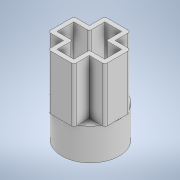
# Autodesk Inventor part: servo-axle-adapter-1-2
Saved by Autodesk Inventor 2020 (Build 240168000, 168)
## iProperties
Created: 2023-03-22
Part Number: servo-axle-adapter-1-2
Material: Generic
Document SubType Name: Modeling
Designer: 22hamfri
Density: 1 g/cm^3
Appearance: Default
Author: 22hamfri
Autodesk Inventor part; units mm, degrees
ref_plane "YZ Plane" through (0, 0, 0) normal (1, 0, 0) x (0, 1, 0)
ref_plane "XZ Plane" through (0, 0, 0) normal (0, 1, 0) x (-1, 0, 0)
ref_plane "XY Plane" through (0, 0, 0) normal (0, 0, 1) x (1, 0, 0)
sketch "Sketch1" plane through (0, 0, 0) normal (0, 1, 0) x (-1, 0, 0)
  circle A0 centre (0, 0) radius 2.6478
  line L0 (2.6478, 0) -> (2.4043, 0.3165)
  line L1 (2.6478, 0) -> (0, 0)
  line L2 (2.6478, 0) -> (2.4043, -0.3165)
  line L3 (2.5576, 0.6853) -> (2.2404, 0.928)
  line L4 (2.5576, 0.6853) -> (2.4043, 0.3165)
  line L5 (2.293, 1.3239) -> (1.9239, 1.4762)
  line L6 (2.293, 1.3239) -> (2.2404, 0.928)
  line L7 (1.8723, 1.8723) -> (1.4762, 1.9239)
  line L8 (1.8723, 1.8723) -> (1.9239, 1.4762)
  line L9 (1.3239, 2.293) -> (0.928, 2.2404)
  line L10 (1.3239, 2.293) -> (1.4762, 1.9239)
  line L11 (0.6853, 2.5576) -> (0.3165, 2.4043)
  line L12 (0.6853, 2.5576) -> (0.928, 2.2404)
  line L13 (0, 2.6478) -> (-0.3165, 2.4043)
  line L14 (0, 2.6478) -> (0.3165, 2.4043)
  line L15 (-0.6853, 2.5576) -> (-0.928, 2.2404)
  line L16 (-0.6853, 2.5576) -> (-0.3165, 2.4043)
  line L17 (-1.3239, 2.293) -> (-1.4762, 1.9239)
  line L18 (-1.3239, 2.293) -> (-0.928, 2.2404)
  line L19 (-1.8723, 1.8723) -> (-1.9239, 1.4762)
  line L20 (-1.8723, 1.8723) -> (-1.4762, 1.9239)
  line L21 (-2.293, 1.3239) -> (-2.2404, 0.928)
  line L22 (-2.293, 1.3239) -> (-1.9239, 1.4762)
  line L23 (-2.5576, 0.6853) -> (-2.4043, 0.3165)
  line L24 (-2.5576, 0.6853) -> (-2.2404, 0.928)
  line L25 (-2.6478, 0) -> (-2.4043, -0.3165)
  line L26 (-2.6478, 0) -> (-2.4043, 0.3165)
  line L27 (-2.5576, -0.6853) -> (-2.2404, -0.928)
  line L28 (-2.5576, -0.6853) -> (-2.4043, -0.3165)
  line L29 (-2.293, -1.3239) -> (-1.9239, -1.4762)
  line L30 (-2.293, -1.3239) -> (-2.2404, -0.928)
  line L31 (-1.8723, -1.8723) -> (-1.4762, -1.9239)
  line L32 (-1.8723, -1.8723) -> (-1.9239, -1.4762)
  line L33 (-1.3239, -2.293) -> (-0.928, -2.2404)
  line L34 (-1.3239, -2.293) -> (-1.4762, -1.9239)
  line L35 (-0.6853, -2.5576) -> (-0.3165, -2.4043)
  line L36 (-0.6853, -2.5576) -> (-0.928, -2.2404)
  line L37 (0, -2.6478) -> (0.3165, -2.4043)
  line L38 (0, -2.6478) -> (-0.3165, -2.4043)
  line L39 (0.6853, -2.5576) -> (0.928, -2.2404)
  line L40 (0.6853, -2.5576) -> (0.3165, -2.4043)
  line L41 (1.3239, -2.293) -> (1.4762, -1.9239)
  line L42 (1.3239, -2.293) -> (0.928, -2.2404)
  line L43 (1.8723, -1.8723) -> (1.9239, -1.4762)
  line L44 (1.8723, -1.8723) -> (1.4762, -1.9239)
  line L45 (2.293, -1.3239) -> (2.2404, -0.928)
  line L46 (2.293, -1.3239) -> (1.9239, -1.4762)
  line L47 (2.5576, -0.6853) -> (2.4043, -0.3165)
  line L48 (2.5576, -0.6853) -> (2.2404, -0.928)
  circle A1 centre (0, 0) radius 3.1478
  point P0 (-0.3165, -2.4043)
  point P1 (2.4043, 0.3165)
  dimension "d4" = 360
  dimension "d6" = 104.851
  dimension "d8" = 0.5
  dimension "d33" = 4.85
  constraints: 98 end point, 2 coincident, 1 centre point, 1 horizontal, 1 horizontal alignment, 1 symmetric about line, 123 other
  measures "d6" angle of L2 L0
  measures "d33" distance of L35.end L11.end
extrude "Extrusion1" add sketch "Sketch1" along normal blind 3 contours L0 L4 A0 | A0 L47 L2 | L3 L6 A0 | A0 L45 L48 | L5 L8 A0 | A0 L43 L46 | L7 L10 A0 | A0 L41 L44 | L9 L12 A0 | A0 L39 L42 | L11 L14 A0 | A0 L37 L40 | L13 L16 A0 | A0 L35 L38 | L15 L18 A0 | A0 L33 L36 | L17 L20 A0 | A0 L31 L34 | L19 L22 A0 | A0 L29 L32 | L21 L24 A0 | A0 L27 L30 | L23 L26 A0 | A0 L25 L28 | A1
sketch "Sketch2" plane through (0, 3, 0) normal (0, 1, 0) x (1, 0, 0)
  circle A0 centre (0, 0) radius 3.1478 projected
  line L0 (1.3239, -2.293) -> (0.928, -2.2404) projected
  line L1 (0.928, -2.2404) -> (0.6853, -2.5576) projected
  line L2 (0.6853, -2.5576) -> (0.3165, -2.4043) projected
  line L3 (0.3165, -2.4043) -> (0, -2.6478) projected
  line L4 (0, -2.6478) -> (-0.3165, -2.4043) projected
  line L5 (-0.3165, -2.4043) -> (-0.6853, -2.5576) projected
  line L6 (-0.6853, -2.5576) -> (-0.928, -2.2404) projected
  line L7 (-0.928, -2.2404) -> (-1.3239, -2.293) projected
  line L8 (-1.3239, -2.293) -> (-1.4762, -1.9239) projected
  line L9 (-1.4762, -1.9239) -> (-1.8723, -1.8723) projected
  line L10 (-1.8723, -1.8723) -> (-1.9239, -1.4762) projected
  line L11 (-1.9239, -1.4762) -> (-2.293, -1.3239) projected
  line L12 (-2.293, -1.3239) -> (-2.2404, -0.928) projected
  line L13 (-2.2404, -0.928) -> (-2.5576, -0.6853) projected
  line L14 (-2.5576, -0.6853) -> (-2.4043, -0.3165) projected
  line L15 (-2.4043, -0.3165) -> (-2.6478, 0) projected
  line L16 (-2.6478, 0) -> (-2.4043, 0.3165) projected
  line L17 (-2.4043, 0.3165) -> (-2.5576, 0.6853) projected
  line L18 (-2.5576, 0.6853) -> (-2.2404, 0.928) projected
  line L19 (-2.2404, 0.928) -> (-2.293, 1.3239) projected
  line L20 (-2.293, 1.3239) -> (-1.9239, 1.4762) projected
  line L21 (-1.9239, 1.4762) -> (-1.8723, 1.8723) projected
  line L22 (-1.8723, 1.8723) -> (-1.4762, 1.9239) projected
  line L23 (-1.4762, 1.9239) -> (-1.3239, 2.293) projected
  line L24 (-1.3239, 2.293) -> (-0.928, 2.2404) projected
  line L25 (-0.928, 2.2404) -> (-0.6853, 2.5576) projected
  line L26 (-0.6853, 2.5576) -> (-0.3165, 2.4043) projected
  line L27 (-0.3165, 2.4043) -> (0, 2.6478) projected
  line L28 (0, 2.6478) -> (0.3165, 2.4043) projected
  line L29 (0.3165, 2.4043) -> (0.6853, 2.5576) projected
  line L30 (0.6853, 2.5576) -> (0.928, 2.2404) projected
  line L31 (0.928, 2.2404) -> (1.3239, 2.293) projected
  line L32 (1.3239, 2.293) -> (1.4762, 1.9239) projected
  line L33 (1.4762, 1.9239) -> (1.8723, 1.8723) projected
  line L34 (1.8723, 1.8723) -> (1.9239, 1.4762) projected
  line L35 (1.9239, 1.4762) -> (2.293, 1.3239) projected
  line L36 (2.293, 1.3239) -> (2.2404, 0.928) projected
  line L37 (2.2404, 0.928) -> (2.5576, 0.6853) projected
  line L38 (2.5576, 0.6853) -> (2.4043, 0.3165) projected
  line L39 (2.4043, 0.3165) -> (2.6478, 0) projected
  line L40 (2.6478, 0) -> (2.4043, -0.3165) projected
  line L41 (2.4043, -0.3165) -> (2.5576, -0.6853) projected
  line L42 (2.5576, -0.6853) -> (2.2404, -0.928) projected
  line L43 (2.2404, -0.928) -> (2.293, -1.3239) projected
  line L44 (2.293, -1.3239) -> (1.9239, -1.4762) projected
  line L45 (1.9239, -1.4762) -> (1.8723, -1.8723) projected
  line L46 (1.8723, -1.8723) -> (1.4762, -1.9239) projected
  line L47 (1.4762, -1.9239) -> (1.3239, -2.293) projected
extrude "Extrusion2" add sketch "Sketch2" along normal blind 0.5 contours A0 | L0 L1 L2 L3 L4 L5 L6 L7 L8 L9 L10 L11 L12 L13 L14 L15 L16 L17 L18 L19 L20 L21 L22 L23 L24 L25 L26 L27 L28 L29 L30 L31 L32 L33 L34 L35 L36 L37 L38 L39 L40 L41 L42 L43 L44 L45 L46 L47
sketch "Sketch3" plane through (0, 3.5, 0) normal (0, 1, 0) x (1, 0, 0)
  line L0 (2.625, -1.05) -> (-2.625, -1.05)
  line L1 (-2.625, -1.05) -> (-2.625, 0.8)
  line L2 (-2.625, 0.8) -> (2.625, 0.8)
  line L3 (2.625, 0.8) -> (2.625, -1.05)
  line L4 (2.625, -1.05) -> (-2.625, 0.8) construction
  line L5 (-2.625, -1.05) -> (2.625, 0.8) construction
  line L6 (-0.925, -2.75) -> (-0.925, 2.5)
  line L7 (-0.925, 2.5) -> (0.925, 2.5)
  line L8 (0.925, 2.5) -> (0.925, -2.75)
  line L9 (0.925, -2.75) -> (-0.925, -2.75)
  line L10 (-0.925, -2.75) -> (0.925, 2.5) construction
  line L11 (-0.925, 2.5) -> (0.925, -2.75) construction
  line L12 (-3.125, -1.55) -> (3.125, -1.55)
  line L13 (3.125, -1.55) -> (3.125, 1.3)
  line L14 (3.125, 1.3) -> (-3.125, 1.3)
  line L15 (-3.125, 1.3) -> (-3.125, -1.55)
  line L16 (-1.425, 3) -> (-1.425, -3.25)
  line L17 (-1.425, -3.25) -> (1.425, -3.25)
  line L18 (1.425, -3.25) -> (1.425, 3)
  line L19 (1.425, 3) -> (-1.425, 3)
  point P0 (0, -0.125)
  point P1 (0.925, -1.05)
  point P2 (-0.925, -1.05)
  point P3 (-0.925, 0.8)
  point P4 (0.925, 0.8)
  point P5 (1.425, -1.55)
  point P6 (1.425, 1.3)
  point P7 (-1.425, 1.3)
  point P8 (-1.425, -1.55)
  dimension "d17" = 5.25
  dimension "d15" = 5.25
  dimension "d18" = 1.85
  dimension "d16" = 1.85
  dimension "d13" = 0.5
  dimension "d14" = 0.5
  constraints: 40 end point, 8 parallel, 4 midpoint, 4 perpendicular, 1 horizontal, 1 vertical, 6 other
  measures "d17" distance between parallel lines of L3 L1
  measures "d15" distance between parallel lines of L7 L9
  measures "d18" distance between parallel lines of L2 L0
  measures "d16" distance between parallel lines of L8 L6
  measures "d13" distance between parallel lines of L19 L7
  measures "d14" distance between parallel lines of L13 L3
extrude "Extrusion3" add sketch "Sketch3" along normal blind 6 contours L3 L2 L18 L14 L13 L12 L0 | L18 L12 L8 L0 | L18 L17 L16 L12 L6 L9 L8 | L2 L8 L14 L18 | L6 L12 L16 L0 | L14 L8 L7 L6 L16 L19 L18 | L16 L12 L15 L14 L2 L1 L0 | L2 L16 L14 L6
fillet "Fillet1" radius 0.3 8 edges at (1.425, 6.5, 3.25) (3.125, 6.5, 1.55) (3.125, 6.5, -1.3) (1.425, 6.5, -3) (-1.425, 6.5, -3) (-3.125, 6.5, -1.3) (-3.125, 6.5, 1.55) (-1.425, 6.5, 3.25)
fillet "Fillet2" radius 0.2 4 edges at (0.925, 6.5, 1.05) (-0.925, 6.5, 1.05) (-0.925, 6.5, -0.8) (0.925, 6.5, -0.8)
sketch "Sketch5" plane through (0, 3.5, 0) normal (0, 1, 0) x (1, 0, 0)
  line L0 (0.925, 2.5) -> (-0.925, 2.5) projected
  line L1 (-0.925, 2.5) -> (-0.925, 1) projected
  arc A0 (-1.125, 0.8) -> (-0.925, 1) centre (-1.125, 1) ccw projected
  line L2 (-1.125, 0.8) -> (-2.625, 0.8) projected
  line L3 (-2.625, 0.8) -> (-2.625, -1.05) projected
  line L4 (-2.625, -1.05) -> (-1.125, -1.05) projected
  arc A1 (-0.925, -1.25) -> (-1.125, -1.05) centre (-1.125, -1.25) ccw projected
  line L5 (-0.925, -1.25) -> (-0.925, -2.75) projected
  line L6 (-0.925, -2.75) -> (0.925, -2.75) projected
  line L7 (0.925, -2.75) -> (0.925, -1.25) projected
  arc A2 (1.125, -1.05) -> (0.925, -1.25) centre (1.125, -1.25) ccw projected
  line L8 (1.125, -1.05) -> (2.625, -1.05) projected
  line L9 (2.625, -1.05) -> (2.625, 0.8) projected
  line L10 (2.625, 0.8) -> (1.125, 0.8) projected
  arc A3 (0.925, 1) -> (1.125, 0.8) centre (1.125, 1) ccw projected
  line L11 (0.925, 1) -> (0.925, 2.5) projected
  line L12 (1.4762, -1.9239) -> (1.3239, -2.293) projected
  line L13 (1.3239, -2.293) -> (0.928, -2.2404) projected
  line L14 (0.928, -2.2404) -> (0.6853, -2.5576) projected
  line L15 (0.6853, -2.5576) -> (0.3165, -2.4043) projected
  line L16 (0.3165, -2.4043) -> (0, -2.6478) projected
  line L17 (0, -2.6478) -> (-0.3165, -2.4043) projected
  line L18 (-0.3165, -2.4043) -> (-0.6853, -2.5576) projected
  line L19 (-0.6853, -2.5576) -> (-0.928, -2.2404) projected
  line L20 (-0.928, -2.2404) -> (-1.3239, -2.293) projected
  line L21 (-1.3239, -2.293) -> (-1.4762, -1.9239) projected
  line L22 (-1.4762, -1.9239) -> (-1.8723, -1.8723) projected
  line L23 (-1.8723, -1.8723) -> (-1.9239, -1.4762) projected
  line L24 (-1.9239, -1.4762) -> (-2.293, -1.3239) projected
  line L25 (-2.293, -1.3239) -> (-2.2404, -0.928) projected
  line L26 (-2.2404, -0.928) -> (-2.5576, -0.6853) projected
  line L27 (-2.5576, -0.6853) -> (-2.4043, -0.3165) projected
  line L28 (-2.4043, -0.3165) -> (-2.6478, 0) projected
  line L29 (-2.6478, 0) -> (-2.4043, 0.3165) projected
  line L30 (-2.4043, 0.3165) -> (-2.5576, 0.6853) projected
  line L31 (-2.5576, 0.6853) -> (-2.2404, 0.928) projected
  line L32 (-2.2404, 0.928) -> (-2.293, 1.3239) projected
  line L33 (-2.293, 1.3239) -> (-1.9239, 1.4762) projected
  line L34 (-1.9239, 1.4762) -> (-1.8723, 1.8723) projected
  line L35 (-1.8723, 1.8723) -> (-1.4762, 1.9239) projected
  line L36 (-1.4762, 1.9239) -> (-1.3239, 2.293) projected
  line L37 (-1.3239, 2.293) -> (-0.928, 2.2404) projected
  line L38 (-0.928, 2.2404) -> (-0.6853, 2.5576) projected
  line L39 (-0.6853, 2.5576) -> (-0.3165, 2.4043) projected
  line L40 (-0.3165, 2.4043) -> (0, 2.6478) projected
  line L41 (0, 2.6478) -> (0.3165, 2.4043) projected
  line L42 (0.3165, 2.4043) -> (0.6853, 2.5576) projected
  line L43 (0.6853, 2.5576) -> (0.928, 2.2404) projected
  line L44 (0.928, 2.2404) -> (1.3239, 2.293) projected
  line L45 (1.3239, 2.293) -> (1.4762, 1.9239) projected
  line L46 (1.4762, 1.9239) -> (1.8723, 1.8723) projected
  line L47 (1.8723, 1.8723) -> (1.9239, 1.4762) projected
  line L48 (1.9239, 1.4762) -> (2.293, 1.3239) projected
  line L49 (2.293, 1.3239) -> (2.2404, 0.928) projected
  line L50 (2.2404, 0.928) -> (2.5576, 0.6853) projected
  line L51 (2.5576, 0.6853) -> (2.4043, 0.3165) projected
  line L52 (2.4043, 0.3165) -> (2.6478, 0) projected
  line L53 (2.6478, 0) -> (2.4043, -0.3165) projected
  line L54 (2.4043, -0.3165) -> (2.5576, -0.6853) projected
  line L55 (2.5576, -0.6853) -> (2.2404, -0.928) projected
  line L56 (2.2404, -0.928) -> (2.293, -1.3239) projected
  line L57 (2.293, -1.3239) -> (1.9239, -1.4762) projected
  line L58 (1.9239, -1.4762) -> (1.8723, -1.8723) projected
  line L59 (1.8723, -1.8723) -> (1.4762, -1.9239) projected
  line L60 (-0.925, 2.5) -> (-0.925, 1) projected
  line L61 (-0.925, 2.2404) -> (0.925, 2.2404)
  line L62 (0.925, 1) -> (0.925, 2.5) projected
  line L63 (2.625, 0.8) -> (1.125, 0.8) projected
  line L64 (2.2404, 0.8) -> (2.2404, -1.05)
  line L65 (1.125, -1.05) -> (2.625, -1.05) projected
  line L66 (-0.925, -1.25) -> (-0.925, -2.75) projected
  line L67 (-0.925, -2.2404) -> (0.925, -2.2404)
  line L68 (0.925, -2.75) -> (0.925, -1.25) projected
  line L69 (-2.625, -1.05) -> (-1.125, -1.05) projected
  line L70 (-2.2404, -1.05) -> (-2.2404, 0.8)
  line L71 (-1.125, 0.8) -> (-2.625, 0.8) projected
  point P0 (0, 0)
  constraints: 12 point on line, 8 end point, 3 perpendicular, 1 horizontal
extrude "Extrusion5" cut sketch "Sketch5" against normal through all contours L11 A3 L10 L64 L8 A2 L7 L67 L5 A1 L4 L70 L2 A0 L1 L61
equation "\"d15\" = d17"
equation "\"d16\" = d18"
equation "\"d14\" = d13"
body "Solid1"
